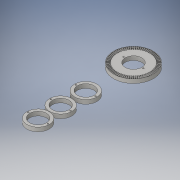
# Autodesk Inventor part: ENCODER_HERE
Saved by Autodesk Inventor 2016 (Build 200138000, 138)
## iProperties
Created: 2018-01-19
Part Number: ENCODER_HERE
Material: Generic
Document SubType Name: Modeling
Designer: student
Density: 1 g/cm^3
Appearance: Default
Author: student
Autodesk Inventor part; units mm, degrees
ref_plane "YZ Plane" through (0, 0, 0) normal (1, 0, 0) x (0, 1, 0)
ref_plane "XZ Plane" through (0, 0, 0) normal (0, 1, 0) x (-1, 0, 0)
ref_plane "XY Plane" through (0, 0, 0) normal (0, 0, 1) x (1, 0, 0)
sketch "Sketch1" plane through (0, 0, 0) normal (0, 1, 0) x (-1, 0, 0)
  circle A0 centre (0, 0) radius 25.4
  circle A1 centre (0, 0) radius 10.5918
  line L0 (-24.8267, 0) -> (-24.8267, 0.5)
  line L1 (-24.8267, 0) -> (-24.8267, -0.5)
  line L2 (-20.6267, 0) -> (-20.6183, 0.4152)
  line L3 (-20.6267, 0) -> (-20.635, -0.4156)
  line L4 (-24.8267, -0.5) -> (-20.635, -0.4156)
  line L5 (-24.8267, 0.5) -> (-20.6183, 0.4152)
  line L6 (-20.5631, -1.6184) -> (-20.5873, -1.2037)
  line L7 (-20.5631, -1.6184) -> (-20.5388, -2.0333)
  line L8 (-24.7894, -1.4494) -> (-20.5873, -1.2037)
  line L9 (-24.7109, -2.4463) -> (-20.5388, -2.0333)
  line L10 (-24.7501, -1.9479) -> (-24.7894, -1.4494)
  line L11 (-24.7501, -1.9479) -> (-24.7109, -2.4463)
  line L12 (-20.3727, -3.2267) -> (-20.4294, -2.8153)
  line L13 (-20.3727, -3.2267) -> (-20.316, -3.6385)
  line L14 (-24.5992, -3.3899) -> (-20.4294, -2.8153)
  line L15 (-24.4428, -4.3776) -> (-20.316, -3.6385)
  line L16 (-24.521, -3.8837) -> (-24.5992, -3.3899)
  line L17 (-24.521, -3.8837) -> (-24.4428, -4.3776)
  line L18 (-20.0568, -4.8152) -> (-20.1456, -4.4095)
  line L19 (-20.0568, -4.8152) -> (-19.9679, -5.2213)
  line L20 (-24.2574, -5.3095) -> (-20.1456, -4.4095)
  line L21 (-24.024, -6.2819) -> (-19.9679, -5.2213)
  line L22 (-24.1407, -5.7957) -> (-24.2574, -5.3095)
  line L23 (-24.1407, -5.7957) -> (-24.024, -6.2819)
  line L24 (-19.6171, -6.374) -> (-19.7375, -5.9765)
  line L25 (-19.6171, -6.374) -> (-19.4967, -6.7718)
  line L26 (-23.7661, -7.1963) -> (-19.7375, -5.9765)
  line L27 (-23.4571, -8.1474) -> (-19.4967, -6.7718)
  line L28 (-23.6116, -7.6719) -> (-23.7661, -7.1963)
  line L29 (-23.6116, -7.6719) -> (-23.4571, -8.1474)
  line L30 (-19.0566, -7.8935) -> (-19.2077, -7.5067)
  line L31 (-19.0566, -7.8935) -> (-18.9053, -8.2806)
  line L32 (-23.1282, -9.0388) -> (-19.2077, -7.5067)
  line L33 (-22.7455, -9.9627) -> (-18.9053, -8.2806)
  line L34 (-22.9369, -9.5008) -> (-23.1282, -9.0388)
  line L35 (-22.9369, -9.5008) -> (-22.7455, -9.9627)
  line L36 (-18.3785, -9.3643) -> (-18.5596, -8.9905)
  line L37 (-18.3785, -9.3643) -> (-18.1973, -9.7384)
  line L38 (-22.3477, -10.8256) -> (-18.5596, -8.9905)
  line L39 (-21.8937, -11.7166) -> (-18.1973, -9.7384)
  line L40 (-22.1207, -11.2711) -> (-22.3477, -10.8256)
  line L41 (-22.1207, -11.2711) -> (-21.8937, -11.7166)
  line L42 (-17.5871, -10.7774) -> (-17.797, -10.419)
  line L43 (-17.5871, -10.7774) -> (-17.3771, -11.1361)
  line L44 (-21.4295, -12.5456) -> (-17.797, -10.419)
  line L45 (-20.907, -13.3982) -> (-17.3771, -11.1361)
  line L46 (-21.1682, -12.9719) -> (-21.4295, -12.5456)
  line L47 (-21.1682, -12.9719) -> (-20.907, -13.3982)
  line L48 (-16.6873, -12.1241) -> (-16.9246, -11.7832)
  line L49 (-16.6873, -12.1241) -> (-16.4498, -12.4652)
  line L50 (-20.3791, -14.1882) -> (-16.9246, -11.7832)
  line L51 (-19.7913, -14.9973) -> (-16.4498, -12.4652)
  line L52 (-20.0852, -14.5928) -> (-20.3791, -14.1882)
  line L53 (-20.0852, -14.5928) -> (-19.7913, -14.9973)
  line L54 (-15.6846, -13.396) -> (-15.948, -13.0748)
  line L55 (-15.6846, -13.396) -> (-15.4211, -13.7174)
  line L56 (-19.2031, -15.7434) -> (-15.948, -13.0748)
  line L57 (-18.5536, -16.5038) -> (-15.4211, -13.7174)
  line L58 (-18.8784, -16.1236) -> (-19.2031, -15.7434)
  line L59 (-18.8784, -16.1236) -> (-18.5536, -16.5038)
  line L60 (-14.5853, -14.5853) -> (-14.873, -14.2857)
  line L61 (-14.5853, -14.5853) -> (-14.2973, -14.885)
  line L62 (-17.9087, -17.2016) -> (-14.873, -14.2857)
  line L63 (-17.2016, -17.9087) -> (-14.2973, -14.885)
  line L64 (-17.5551, -17.5551) -> (-17.9087, -17.2016)
  line L65 (-17.5551, -17.5551) -> (-17.2016, -17.9087)
  line L66 (-13.396, -15.6846) -> (-13.7063, -15.4086)
  line L67 (-13.396, -15.6846) -> (-13.0854, -15.9609)
  line L68 (-16.5038, -18.5536) -> (-13.7063, -15.4086)
  line L69 (-15.7434, -19.2031) -> (-13.0854, -15.9609)
  line L70 (-16.1236, -18.8784) -> (-16.5038, -18.5536)
  line L71 (-16.1236, -18.8784) -> (-15.7434, -19.2031)
  line L72 (-12.1241, -16.6873) -> (-12.4551, -16.4365)
  line L73 (-12.1241, -16.6873) -> (-11.7928, -16.9384)
  line L74 (-14.9973, -19.7913) -> (-12.4551, -16.4365)
  line L75 (-14.1882, -20.3791) -> (-11.7928, -16.9384)
  line L76 (-14.5928, -20.0852) -> (-14.9973, -19.7913)
  line L77 (-14.5928, -20.0852) -> (-14.1882, -20.3791)
  line L78 (-10.7774, -17.5871) -> (-11.1271, -17.363)
  line L79 (-10.7774, -17.5871) -> (-10.4274, -17.8114)
  line L80 (-13.3982, -20.907) -> (-11.1271, -17.363)
  line L81 (-12.5456, -21.4295) -> (-10.4274, -17.8114)
  line L82 (-12.9719, -21.1682) -> (-13.3982, -20.907)
  line L83 (-12.9719, -21.1682) -> (-12.5456, -21.4295)
  line L84 (-9.3643, -18.3785) -> (-9.7305, -18.1825)
  line L85 (-9.3643, -18.3785) -> (-8.9978, -18.5746)
  line L86 (-11.7166, -21.8937) -> (-9.7305, -18.1825)
  line L87 (-10.8256, -22.3477) -> (-8.9978, -18.5746)
  line L88 (-11.2711, -22.1207) -> (-11.7166, -21.8937)
  line L89 (-11.2711, -22.1207) -> (-10.8256, -22.3477)
  line L90 (-7.8935, -19.0566) -> (-8.2739, -18.8899)
  line L91 (-7.8935, -19.0566) -> (-7.5127, -19.2233)
  line L92 (-9.9627, -22.7455) -> (-8.2739, -18.8899)
  line L93 (-9.0388, -23.1282) -> (-7.5127, -19.2233)
  line L94 (-9.5008, -22.9369) -> (-9.9627, -22.7455)
  line L95 (-9.5008, -22.9369) -> (-9.0388, -23.1282)
  line L96 (-6.374, -19.6171) -> (-6.7663, -19.4809)
  line L97 (-6.374, -19.6171) -> (-5.9813, -19.7535)
  line L98 (-8.1474, -23.4571) -> (-6.7663, -19.4809)
  line L99 (-7.1963, -23.7661) -> (-5.9813, -19.7535)
  line L100 (-7.6719, -23.6116) -> (-8.1474, -23.4571)
  line L101 (-7.6719, -23.6116) -> (-7.1963, -23.7661)
  line L102 (-4.8152, -20.0568) -> (-5.217, -19.9517)
  line L103 (-4.8152, -20.0568) -> (-4.4131, -20.1619)
  line L104 (-6.2819, -24.024) -> (-5.217, -19.9517)
  line L105 (-5.3095, -24.2574) -> (-4.4131, -20.1619)
  line L106 (-5.7957, -24.1407) -> (-6.2819, -24.024)
  line L107 (-5.7957, -24.1407) -> (-5.3095, -24.2574)
  line L108 (-3.2267, -20.3727) -> (-3.6355, -20.2995)
  line L109 (-3.2267, -20.3727) -> (-2.8176, -20.446)
  line L110 (-4.3776, -24.4428) -> (-3.6355, -20.2995)
  line L111 (-3.3899, -24.5992) -> (-2.8176, -20.446)
  line L112 (-3.8837, -24.521) -> (-4.3776, -24.4428)
  line L113 (-3.8837, -24.521) -> (-3.3899, -24.5992)
  line L114 (-1.6184, -20.5631) -> (-2.0317, -20.5222)
  line L115 (-1.6184, -20.5631) -> (-1.2047, -20.604)
  line L116 (-2.4463, -24.7109) -> (-2.0317, -20.5222)
  line L117 (-1.4494, -24.7894) -> (-1.2047, -20.604)
  line L118 (-1.9479, -24.7501) -> (-2.4463, -24.7109)
  line L119 (-1.9479, -24.7501) -> (-1.4494, -24.7894)
  line L120 (0, -20.6267) -> (-0.4152, -20.6183)
  line L121 (0, -20.6267) -> (0.4156, -20.635)
  line L122 (-0.5, -24.8267) -> (-0.4152, -20.6183)
  line L123 (0.5, -24.8267) -> (0.4156, -20.635)
  line L124 (0, -24.8267) -> (-0.5, -24.8267)
  line L125 (0, -24.8267) -> (0.5, -24.8267)
  line L126 (1.6184, -20.5631) -> (1.2037, -20.5873)
  line L127 (1.6184, -20.5631) -> (2.0333, -20.5388)
  line L128 (1.4494, -24.7894) -> (1.2037, -20.5873)
  line L129 (2.4463, -24.7109) -> (2.0333, -20.5388)
  line L130 (1.9479, -24.7501) -> (1.4494, -24.7894)
  line L131 (1.9479, -24.7501) -> (2.4463, -24.7109)
  line L132 (3.2267, -20.3727) -> (2.8153, -20.4294)
  line L133 (3.2267, -20.3727) -> (3.6385, -20.316)
  line L134 (3.3899, -24.5992) -> (2.8153, -20.4294)
  line L135 (4.3776, -24.4428) -> (3.6385, -20.316)
  line L136 (3.8837, -24.521) -> (3.3899, -24.5992)
  line L137 (3.8837, -24.521) -> (4.3776, -24.4428)
  line L138 (4.8152, -20.0568) -> (4.4095, -20.1456)
  line L139 (4.8152, -20.0568) -> (5.2213, -19.9679)
  line L140 (5.3095, -24.2574) -> (4.4095, -20.1456)
  line L141 (6.2819, -24.024) -> (5.2213, -19.9679)
  line L142 (5.7957, -24.1407) -> (5.3095, -24.2574)
  line L143 (5.7957, -24.1407) -> (6.2819, -24.024)
  line L144 (6.374, -19.6171) -> (5.9765, -19.7375)
  line L145 (6.374, -19.6171) -> (6.7718, -19.4967)
  line L146 (7.1963, -23.7661) -> (5.9765, -19.7375)
  line L147 (8.1474, -23.4571) -> (6.7718, -19.4967)
  line L148 (7.6719, -23.6116) -> (7.1963, -23.7661)
  line L149 (7.6719, -23.6116) -> (8.1474, -23.4571)
  line L150 (7.8935, -19.0566) -> (7.5067, -19.2077)
  line L151 (7.8935, -19.0566) -> (8.2806, -18.9053)
  line L152 (9.0388, -23.1282) -> (7.5067, -19.2077)
  line L153 (9.9627, -22.7455) -> (8.2806, -18.9053)
  line L154 (9.5008, -22.9369) -> (9.0388, -23.1282)
  line L155 (9.5008, -22.9369) -> (9.9627, -22.7455)
  line L156 (9.3643, -18.3785) -> (8.9905, -18.5596)
  line L157 (9.3643, -18.3785) -> (9.7384, -18.1973)
  line L158 (10.8256, -22.3477) -> (8.9905, -18.5596)
  line L159 (11.7166, -21.8937) -> (9.7384, -18.1973)
  line L160 (11.2711, -22.1207) -> (10.8256, -22.3477)
  line L161 (11.2711, -22.1207) -> (11.7166, -21.8937)
  line L162 (10.7774, -17.5871) -> (10.419, -17.797)
  line L163 (10.7774, -17.5871) -> (11.1361, -17.3771)
  line L164 (12.5456, -21.4295) -> (10.419, -17.797)
  line L165 (13.3982, -20.907) -> (11.1361, -17.3771)
  line L166 (12.9719, -21.1682) -> (12.5456, -21.4295)
  line L167 (12.9719, -21.1682) -> (13.3982, -20.907)
  line L168 (12.1241, -16.6873) -> (11.7832, -16.9246)
  line L169 (12.1241, -16.6873) -> (12.4652, -16.4498)
  line L170 (14.1882, -20.3791) -> (11.7832, -16.9246)
  line L171 (14.9973, -19.7913) -> (12.4652, -16.4498)
  line L172 (14.5928, -20.0852) -> (14.1882, -20.3791)
  line L173 (14.5928, -20.0852) -> (14.9973, -19.7913)
  line L174 (13.396, -15.6846) -> (13.0748, -15.948)
  line L175 (13.396, -15.6846) -> (13.7174, -15.4211)
  line L176 (15.7434, -19.2031) -> (13.0748, -15.948)
  line L177 (16.5038, -18.5536) -> (13.7174, -15.4211)
  line L178 (16.1236, -18.8784) -> (15.7434, -19.2031)
  line L179 (16.1236, -18.8784) -> (16.5038, -18.5536)
  line L180 (14.5853, -14.5853) -> (14.2857, -14.873)
  line L181 (14.5853, -14.5853) -> (14.885, -14.2973)
  line L182 (17.2016, -17.9087) -> (14.2857, -14.873)
  line L183 (17.9087, -17.2016) -> (14.885, -14.2973)
  line L184 (17.5551, -17.5551) -> (17.2016, -17.9087)
  line L185 (17.5551, -17.5551) -> (17.9087, -17.2016)
  line L186 (15.6846, -13.396) -> (15.4086, -13.7063)
  line L187 (15.6846, -13.396) -> (15.9609, -13.0854)
  line L188 (18.5536, -16.5038) -> (15.4086, -13.7063)
  line L189 (19.2031, -15.7434) -> (15.9609, -13.0854)
  line L190 (18.8784, -16.1236) -> (18.5536, -16.5038)
  line L191 (18.8784, -16.1236) -> (19.2031, -15.7434)
  line L192 (16.6873, -12.1241) -> (16.4365, -12.4551)
  line L193 (16.6873, -12.1241) -> (16.9384, -11.7928)
  line L194 (19.7913, -14.9973) -> (16.4365, -12.4551)
  line L195 (20.3791, -14.1882) -> (16.9384, -11.7928)
  line L196 (20.0852, -14.5928) -> (19.7913, -14.9973)
  line L197 (20.0852, -14.5928) -> (20.3791, -14.1882)
  line L198 (17.5871, -10.7774) -> (17.363, -11.1271)
  line L199 (17.5871, -10.7774) -> (17.8114, -10.4274)
  line L200 (20.907, -13.3982) -> (17.363, -11.1271)
  line L201 (21.4295, -12.5456) -> (17.8114, -10.4274)
  line L202 (21.1682, -12.9719) -> (20.907, -13.3982)
  line L203 (21.1682, -12.9719) -> (21.4295, -12.5456)
  line L204 (18.3785, -9.3643) -> (18.1825, -9.7305)
  line L205 (18.3785, -9.3643) -> (18.5746, -8.9978)
  line L206 (21.8937, -11.7166) -> (18.1825, -9.7305)
  line L207 (22.3477, -10.8256) -> (18.5746, -8.9978)
  line L208 (22.1207, -11.2711) -> (21.8937, -11.7166)
  line L209 (22.1207, -11.2711) -> (22.3477, -10.8256)
  line L210 (19.0566, -7.8935) -> (18.8899, -8.2739)
  line L211 (19.0566, -7.8935) -> (19.2233, -7.5127)
  line L212 (22.7455, -9.9627) -> (18.8899, -8.2739)
  line L213 (23.1282, -9.0388) -> (19.2233, -7.5127)
  line L214 (22.9369, -9.5008) -> (22.7455, -9.9627)
  line L215 (22.9369, -9.5008) -> (23.1282, -9.0388)
  line L216 (19.6171, -6.374) -> (19.4809, -6.7663)
  line L217 (19.6171, -6.374) -> (19.7535, -5.9813)
  line L218 (23.4571, -8.1474) -> (19.4809, -6.7663)
  line L219 (23.7661, -7.1963) -> (19.7535, -5.9813)
  line L220 (23.6116, -7.6719) -> (23.4571, -8.1474)
  line L221 (23.6116, -7.6719) -> (23.7661, -7.1963)
  line L222 (20.0568, -4.8152) -> (19.9517, -5.217)
  line L223 (20.0568, -4.8152) -> (20.1619, -4.4131)
  line L224 (24.024, -6.2819) -> (19.9517, -5.217)
  line L225 (24.2574, -5.3095) -> (20.1619, -4.4131)
  line L226 (24.1407, -5.7957) -> (24.024, -6.2819)
  line L227 (24.1407, -5.7957) -> (24.2574, -5.3095)
  line L228 (20.3727, -3.2267) -> (20.2995, -3.6355)
  line L229 (20.3727, -3.2267) -> (20.446, -2.8176)
  line L230 (24.4428, -4.3776) -> (20.2995, -3.6355)
  line L231 (24.5992, -3.3899) -> (20.446, -2.8176)
  line L232 (24.521, -3.8837) -> (24.4428, -4.3776)
  line L233 (24.521, -3.8837) -> (24.5992, -3.3899)
  line L234 (20.5631, -1.6184) -> (20.5222, -2.0317)
  line L235 (20.5631, -1.6184) -> (20.604, -1.2047)
  line L236 (24.7109, -2.4463) -> (20.5222, -2.0317)
  line L237 (24.7894, -1.4494) -> (20.604, -1.2047)
  line L238 (24.7501, -1.9479) -> (24.7109, -2.4463)
  line L239 (24.7501, -1.9479) -> (24.7894, -1.4494)
  line L240 (20.6267, 0) -> (20.6183, -0.4152)
  line L241 (20.6267, 0) -> (20.635, 0.4156)
  line L242 (24.8267, -0.5) -> (20.6183, -0.4152)
  line L243 (24.8267, 0.5) -> (20.635, 0.4156)
  line L244 (24.8267, 0) -> (24.8267, -0.5)
  line L245 (24.8267, 0) -> (24.8267, 0.5)
  line L246 (20.5631, 1.6184) -> (20.5873, 1.2037)
  line L247 (20.5631, 1.6184) -> (20.5388, 2.0333)
  line L248 (24.7894, 1.4494) -> (20.5873, 1.2037)
  line L249 (24.7109, 2.4463) -> (20.5388, 2.0333)
  line L250 (24.7501, 1.9479) -> (24.7894, 1.4494)
  line L251 (24.7501, 1.9479) -> (24.7109, 2.4463)
  line L252 (20.3727, 3.2267) -> (20.4294, 2.8153)
  line L253 (20.3727, 3.2267) -> (20.316, 3.6385)
  line L254 (24.5992, 3.3899) -> (20.4294, 2.8153)
  line L255 (24.4428, 4.3776) -> (20.316, 3.6385)
  line L256 (24.521, 3.8837) -> (24.5992, 3.3899)
  line L257 (24.521, 3.8837) -> (24.4428, 4.3776)
  line L258 (20.0568, 4.8152) -> (20.1456, 4.4095)
  line L259 (20.0568, 4.8152) -> (19.9679, 5.2213)
  line L260 (24.2574, 5.3095) -> (20.1456, 4.4095)
  line L261 (24.024, 6.2819) -> (19.9679, 5.2213)
  line L262 (24.1407, 5.7957) -> (24.2574, 5.3095)
  line L263 (24.1407, 5.7957) -> (24.024, 6.2819)
  line L264 (19.6171, 6.374) -> (19.7375, 5.9765)
  line L265 (19.6171, 6.374) -> (19.4967, 6.7718)
  line L266 (23.7661, 7.1963) -> (19.7375, 5.9765)
  line L267 (23.4571, 8.1474) -> (19.4967, 6.7718)
  line L268 (23.6116, 7.6719) -> (23.7661, 7.1963)
  line L269 (23.6116, 7.6719) -> (23.4571, 8.1474)
  line L270 (19.0566, 7.8935) -> (19.2077, 7.5067)
  line L271 (19.0566, 7.8935) -> (18.9053, 8.2806)
  line L272 (23.1282, 9.0388) -> (19.2077, 7.5067)
  line L273 (22.7455, 9.9627) -> (18.9053, 8.2806)
  line L274 (22.9369, 9.5008) -> (23.1282, 9.0388)
  line L275 (22.9369, 9.5008) -> (22.7455, 9.9627)
  line L276 (18.3785, 9.3643) -> (18.5596, 8.9905)
  line L277 (18.3785, 9.3643) -> (18.1973, 9.7384)
  line L278 (22.3477, 10.8256) -> (18.5596, 8.9905)
  line L279 (21.8937, 11.7166) -> (18.1973, 9.7384)
  line L280 (22.1207, 11.2711) -> (22.3477, 10.8256)
  line L281 (22.1207, 11.2711) -> (21.8937, 11.7166)
  line L282 (17.5871, 10.7774) -> (17.797, 10.419)
  line L283 (17.5871, 10.7774) -> (17.3771, 11.1361)
  line L284 (21.4295, 12.5456) -> (17.797, 10.419)
  line L285 (20.907, 13.3982) -> (17.3771, 11.1361)
  line L286 (21.1682, 12.9719) -> (21.4295, 12.5456)
  line L287 (21.1682, 12.9719) -> (20.907, 13.3982)
  line L288 (16.6873, 12.1241) -> (16.9246, 11.7832)
  line L289 (16.6873, 12.1241) -> (16.4498, 12.4652)
  line L290 (20.3791, 14.1882) -> (16.9246, 11.7832)
  line L291 (19.7913, 14.9973) -> (16.4498, 12.4652)
  line L292 (20.0852, 14.5928) -> (20.3791, 14.1882)
  line L293 (20.0852, 14.5928) -> (19.7913, 14.9973)
  line L294 (15.6846, 13.396) -> (15.948, 13.0748)
  line L295 (15.6846, 13.396) -> (15.4211, 13.7174)
  line L296 (19.2031, 15.7434) -> (15.948, 13.0748)
  line L297 (18.5536, 16.5038) -> (15.4211, 13.7174)
  line L298 (18.8784, 16.1236) -> (19.2031, 15.7434)
  line L299 (18.8784, 16.1236) -> (18.5536, 16.5038)
  line L300 (14.5853, 14.5853) -> (14.873, 14.2857)
  line L301 (14.5853, 14.5853) -> (14.2973, 14.885)
  line L302 (17.9087, 17.2016) -> (14.873, 14.2857)
  line L303 (17.2016, 17.9087) -> (14.2973, 14.885)
  line L304 (17.5551, 17.5551) -> (17.9087, 17.2016)
  line L305 (17.5551, 17.5551) -> (17.2016, 17.9087)
  line L306 (13.396, 15.6846) -> (13.7063, 15.4086)
  line L307 (13.396, 15.6846) -> (13.0854, 15.9609)
  line L308 (16.5038, 18.5536) -> (13.7063, 15.4086)
  line L309 (15.7434, 19.2031) -> (13.0854, 15.9609)
  line L310 (16.1236, 18.8784) -> (16.5038, 18.5536)
  line L311 (16.1236, 18.8784) -> (15.7434, 19.2031)
  line L312 (12.1241, 16.6873) -> (12.4551, 16.4365)
  line L313 (12.1241, 16.6873) -> (11.7928, 16.9384)
  line L314 (14.9973, 19.7913) -> (12.4551, 16.4365)
  line L315 (14.1882, 20.3791) -> (11.7928, 16.9384)
  line L316 (14.5928, 20.0852) -> (14.9973, 19.7913)
  line L317 (14.5928, 20.0852) -> (14.1882, 20.3791)
  line L318 (10.7774, 17.5871) -> (11.1271, 17.363)
  line L319 (10.7774, 17.5871) -> (10.4274, 17.8114)
  line L320 (13.3982, 20.907) -> (11.1271, 17.363)
  line L321 (12.5456, 21.4295) -> (10.4274, 17.8114)
  line L322 (12.9719, 21.1682) -> (13.3982, 20.907)
  line L323 (12.9719, 21.1682) -> (12.5456, 21.4295)
  line L324 (9.3643, 18.3785) -> (9.7305, 18.1825)
  line L325 (9.3643, 18.3785) -> (8.9978, 18.5746)
  line L326 (11.7166, 21.8937) -> (9.7305, 18.1825)
  line L327 (10.8256, 22.3477) -> (8.9978, 18.5746)
  line L328 (11.2711, 22.1207) -> (11.7166, 21.8937)
  line L329 (11.2711, 22.1207) -> (10.8256, 22.3477)
  line L330 (7.8935, 19.0566) -> (8.2739, 18.8899)
  line L331 (7.8935, 19.0566) -> (7.5127, 19.2233)
  line L332 (9.9627, 22.7455) -> (8.2739, 18.8899)
  line L333 (9.0388, 23.1282) -> (7.5127, 19.2233)
  line L334 (9.5008, 22.9369) -> (9.9627, 22.7455)
  line L335 (9.5008, 22.9369) -> (9.0388, 23.1282)
  line L336 (6.374, 19.6171) -> (6.7663, 19.4809)
  line L337 (6.374, 19.6171) -> (5.9813, 19.7535)
  line L338 (8.1474, 23.4571) -> (6.7663, 19.4809)
  line L339 (7.1963, 23.7661) -> (5.9813, 19.7535)
  line L340 (7.6719, 23.6116) -> (8.1474, 23.4571)
  line L341 (7.6719, 23.6116) -> (7.1963, 23.7661)
  line L342 (4.8152, 20.0568) -> (5.217, 19.9517)
  line L343 (4.8152, 20.0568) -> (4.4131, 20.1619)
  line L344 (6.2819, 24.024) -> (5.217, 19.9517)
  line L345 (5.3095, 24.2574) -> (4.4131, 20.1619)
  line L346 (5.7957, 24.1407) -> (6.2819, 24.024)
  line L347 (5.7957, 24.1407) -> (5.3095, 24.2574)
  line L348 (3.2267, 20.3727) -> (3.6355, 20.2995)
  line L349 (3.2267, 20.3727) -> (2.8176, 20.446)
  line L350 (4.3776, 24.4428) -> (3.6355, 20.2995)
  line L351 (3.3899, 24.5992) -> (2.8176, 20.446)
  line L352 (3.8837, 24.521) -> (4.3776, 24.4428)
  line L353 (3.8837, 24.521) -> (3.3899, 24.5992)
  line L354 (1.6184, 20.5631) -> (2.0317, 20.5222)
  line L355 (1.6184, 20.5631) -> (1.2047, 20.604)
  line L356 (2.4463, 24.7109) -> (2.0317, 20.5222)
  line L357 (1.4494, 24.7894) -> (1.2047, 20.604)
  line L358 (1.9479, 24.7501) -> (2.4463, 24.7109)
  line L359 (1.9479, 24.7501) -> (1.4494, 24.7894)
  line L360 (0, 20.6267) -> (0.4152, 20.6183)
  line L361 (0, 20.6267) -> (-0.4156, 20.635)
  line L362 (0.5, 24.8267) -> (0.4152, 20.6183)
  line L363 (-0.5, 24.8267) -> (-0.4156, 20.635)
  line L364 (0, 24.8267) -> (0.5, 24.8267)
  line L365 (0, 24.8267) -> (-0.5, 24.8267)
  line L366 (-1.6184, 20.5631) -> (-1.2037, 20.5873)
  line L367 (-1.6184, 20.5631) -> (-2.0333, 20.5388)
  line L368 (-1.4494, 24.7894) -> (-1.2037, 20.5873)
  line L369 (-2.4463, 24.7109) -> (-2.0333, 20.5388)
  line L370 (-1.9479, 24.7501) -> (-1.4494, 24.7894)
  line L371 (-1.9479, 24.7501) -> (-2.4463, 24.7109)
  line L372 (-3.2267, 20.3727) -> (-2.8153, 20.4294)
  line L373 (-3.2267, 20.3727) -> (-3.6385, 20.316)
  line L374 (-3.3899, 24.5992) -> (-2.8153, 20.4294)
  line L375 (-4.3776, 24.4428) -> (-3.6385, 20.316)
  line L376 (-3.8837, 24.521) -> (-3.3899, 24.5992)
  line L377 (-3.8837, 24.521) -> (-4.3776, 24.4428)
  line L378 (-4.8152, 20.0568) -> (-4.4095, 20.1456)
  line L379 (-4.8152, 20.0568) -> (-5.2213, 19.9679)
  line L380 (-5.3095, 24.2574) -> (-4.4095, 20.1456)
  line L381 (-6.2819, 24.024) -> (-5.2213, 19.9679)
  line L382 (-5.7957, 24.1407) -> (-5.3095, 24.2574)
  line L383 (-5.7957, 24.1407) -> (-6.2819, 24.024)
  line L384 (-6.374, 19.6171) -> (-5.9765, 19.7375)
  line L385 (-6.374, 19.6171) -> (-6.7718, 19.4967)
  line L386 (-7.1963, 23.7661) -> (-5.9765, 19.7375)
  line L387 (-8.1474, 23.4571) -> (-6.7718, 19.4967)
  line L388 (-7.6719, 23.6116) -> (-7.1963, 23.7661)
  line L389 (-7.6719, 23.6116) -> (-8.1474, 23.4571)
  line L390 (-7.8935, 19.0566) -> (-7.5067, 19.2077)
  line L391 (-7.8935, 19.0566) -> (-8.2806, 18.9053)
  line L392 (-9.0388, 23.1282) -> (-7.5067, 19.2077)
  line L393 (-9.9627, 22.7455) -> (-8.2806, 18.9053)
  line L394 (-9.5008, 22.9369) -> (-9.0388, 23.1282)
  line L395 (-9.5008, 22.9369) -> (-9.9627, 22.7455)
  line L396 (-9.3643, 18.3785) -> (-8.9905, 18.5596)
  line L397 (-9.3643, 18.3785) -> (-9.7384, 18.1973)
  line L398 (-10.8256, 22.3477) -> (-8.9905, 18.5596)
  line L399 (-11.7166, 21.8937) -> (-9.7384, 18.1973)
  line L400 (-11.2711, 22.1207) -> (-10.8256, 22.3477)
  line L401 (-11.2711, 22.1207) -> (-11.7166, 21.8937)
  line L402 (-10.7774, 17.5871) -> (-10.419, 17.797)
  line L403 (-10.7774, 17.5871) -> (-11.1361, 17.3771)
  line L404 (-12.5456, 21.4295) -> (-10.419, 17.797)
  line L405 (-13.3982, 20.907) -> (-11.1361, 17.3771)
  line L406 (-12.9719, 21.1682) -> (-12.5456, 21.4295)
  line L407 (-12.9719, 21.1682) -> (-13.3982, 20.907)
  line L408 (-12.1241, 16.6873) -> (-11.7832, 16.9246)
  line L409 (-12.1241, 16.6873) -> (-12.4652, 16.4498)
  line L410 (-14.1882, 20.3791) -> (-11.7832, 16.9246)
  line L411 (-14.9973, 19.7913) -> (-12.4652, 16.4498)
  line L412 (-14.5928, 20.0852) -> (-14.1882, 20.3791)
  line L413 (-14.5928, 20.0852) -> (-14.9973, 19.7913)
  line L414 (-13.396, 15.6846) -> (-13.0748, 15.948)
  line L415 (-13.396, 15.6846) -> (-13.7174, 15.4211)
  line L416 (-15.7434, 19.2031) -> (-13.0748, 15.948)
  line L417 (-16.5038, 18.5536) -> (-13.7174, 15.4211)
  line L418 (-16.1236, 18.8784) -> (-15.7434, 19.2031)
  line L419 (-16.1236, 18.8784) -> (-16.5038, 18.5536)
  line L420 (-14.5853, 14.5853) -> (-14.2857, 14.873)
  line L421 (-14.5853, 14.5853) -> (-14.885, 14.2973)
  line L422 (-17.2016, 17.9087) -> (-14.2857, 14.873)
  line L423 (-17.9087, 17.2016) -> (-14.885, 14.2973)
  line L424 (-17.5551, 17.5551) -> (-17.2016, 17.9087)
  line L425 (-17.5551, 17.5551) -> (-17.9087, 17.2016)
  line L426 (-15.6846, 13.396) -> (-15.4086, 13.7063)
  line L427 (-15.6846, 13.396) -> (-15.9609, 13.0854)
  line L428 (-18.5536, 16.5038) -> (-15.4086, 13.7063)
  line L429 (-19.2031, 15.7434) -> (-15.9609, 13.0854)
  line L430 (-18.8784, 16.1236) -> (-18.5536, 16.5038)
  line L431 (-18.8784, 16.1236) -> (-19.2031, 15.7434)
  line L432 (-16.6873, 12.1241) -> (-16.4365, 12.4551)
  line L433 (-16.6873, 12.1241) -> (-16.9384, 11.7928)
  line L434 (-19.7913, 14.9973) -> (-16.4365, 12.4551)
  line L435 (-20.3791, 14.1882) -> (-16.9384, 11.7928)
  line L436 (-20.0852, 14.5928) -> (-19.7913, 14.9973)
  line L437 (-20.0852, 14.5928) -> (-20.3791, 14.1882)
  line L438 (-17.5871, 10.7774) -> (-17.363, 11.1271)
  line L439 (-17.5871, 10.7774) -> (-17.8114, 10.4274)
  line L440 (-20.907, 13.3982) -> (-17.363, 11.1271)
  line L441 (-21.4295, 12.5456) -> (-17.8114, 10.4274)
  line L442 (-21.1682, 12.9719) -> (-20.907, 13.3982)
  line L443 (-21.1682, 12.9719) -> (-21.4295, 12.5456)
  line L444 (-18.3785, 9.3643) -> (-18.1825, 9.7305)
  line L445 (-18.3785, 9.3643) -> (-18.5746, 8.9978)
  line L446 (-21.8937, 11.7166) -> (-18.1825, 9.7305)
  line L447 (-22.3477, 10.8256) -> (-18.5746, 8.9978)
  line L448 (-22.1207, 11.2711) -> (-21.8937, 11.7166)
  line L449 (-22.1207, 11.2711) -> (-22.3477, 10.8256)
  line L450 (-19.0566, 7.8935) -> (-18.8899, 8.2739)
  line L451 (-19.0566, 7.8935) -> (-19.2233, 7.5127)
  line L452 (-22.7455, 9.9627) -> (-18.8899, 8.2739)
  line L453 (-23.1282, 9.0388) -> (-19.2233, 7.5127)
  line L454 (-22.9369, 9.5008) -> (-22.7455, 9.9627)
  line L455 (-22.9369, 9.5008) -> (-23.1282, 9.0388)
  line L456 (-19.6171, 6.374) -> (-19.4809, 6.7663)
  line L457 (-19.6171, 6.374) -> (-19.7535, 5.9813)
  line L458 (-23.4571, 8.1474) -> (-19.4809, 6.7663)
  line L459 (-23.7661, 7.1963) -> (-19.7535, 5.9813)
  line L460 (-23.6116, 7.6719) -> (-23.4571, 8.1474)
  line L461 (-23.6116, 7.6719) -> (-23.7661, 7.1963)
  line L462 (-20.0568, 4.8152) -> (-19.9517, 5.217)
  line L463 (-20.0568, 4.8152) -> (-20.1619, 4.4131)
  line L464 (-24.024, 6.2819) -> (-19.9517, 5.217)
  line L465 (-24.2574, 5.3095) -> (-20.1619, 4.4131)
  line L466 (-24.1407, 5.7957) -> (-24.024, 6.2819)
  line L467 (-24.1407, 5.7957) -> (-24.2574, 5.3095)
  line L468 (-20.3727, 3.2267) -> (-20.2995, 3.6355)
  line L469 (-20.3727, 3.2267) -> (-20.446, 2.8176)
  line L470 (-24.4428, 4.3776) -> (-20.2995, 3.6355)
  line L471 (-24.5992, 3.3899) -> (-20.446, 2.8176)
  line L472 (-24.521, 3.8837) -> (-24.4428, 4.3776)
  line L473 (-24.521, 3.8837) -> (-24.5992, 3.3899)
  line L474 (-20.5631, 1.6184) -> (-20.5222, 2.0317)
  line L475 (-20.5631, 1.6184) -> (-20.604, 1.2047)
  line L476 (-24.7109, 2.4463) -> (-20.5222, 2.0317)
  line L477 (-24.7894, 1.4494) -> (-20.604, 1.2047)
  line L478 (-24.7501, 1.9479) -> (-24.7109, 2.4463)
  line L479 (-24.7501, 1.9479) -> (-24.7894, 1.4494)
  circle A2 centre (12.5456, 0) radius 0.8526
  circle A3 centre (-12.5456, 0) radius 0.8526
  circle A4 centre (0, 0) radius 14.2233
  line L480 (0, 0) -> (-20.6267, 0)
  line L481 (-24.8267, 0) -> (-25.4, 0)
  line L482 (-20.6577, 0) -> (-20.6267, 0)
  circle A5 centre (-0.4152, 61.1951) radius 10.6045
  circle A6 centre (12.1303, 61.1951) radius 0.8526
  circle A7 centre (-12.9608, 61.1951) radius 0.8526
  circle A8 centre (-0.4152, 61.1951) radius 14.2233
  circle A9 centre (-0.4152, 93.1625) radius 10.5918
  circle A10 centre (12.1303, 93.1625) radius 0.8526
  circle A11 centre (-12.9608, 93.1625) radius 0.8526
  circle A12 centre (-0.4152, 93.1625) radius 14.2233
  circle A13 centre (-0.4152, 121.9712) radius 10.6045
  circle A14 centre (12.1303, 121.9712) radius 0.8526
  circle A15 centre (-12.9608, 121.9712) radius 0.8526
  circle A16 centre (-0.4152, 121.9712) radius 14.2233
  dimension "d1" = 21.1836
  dimension "d3" = 0.5
  dimension "d4" = 0.5
  dimension "d7" = 360
  dimension "d11" = 21.209
  dimension "d14" = 21.1836
  dimension "d17" = 21.209
  constraints: 966 end point, 81 point on line, 16 centre point, 5 coincident, 2 horizontal, 2 perpendicular, 1 horizontal alignment, 1 vertical, 963 other
  measures "d1" diameter of A1
  measures "d3" distance of L0.start L0.end
  measures "d4" distance of L0.start L1.end
  measures "d11" diameter of A5
  measures "d14" diameter of A9
  measures "d17" diameter of A13
extrude "Extrusion1" add sketch "Sketch1" along normal blind 5.08 contours A4 | A0 | A8 | A12 | A16
body "Solid1"
